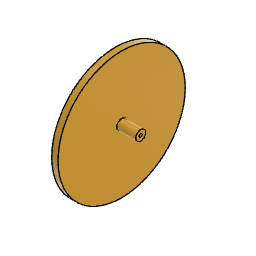
WaterMillWheelRimf3 (Autodesk Fusion 360 design; units mm, degrees)
Autodesk Fusion 360 part; units mm, degrees
sketch "Sketch1" plane through (0, 0, 0) normal (1, 0, 0) x (0, 1, 0)
  circle A0 centre (0, 0) radius 50
  dimension "d1" = 100
  constraint coincident A0.centre origin
  measures "d1" diameter of A0
extrude "Extrude1" add sketch "Sketch1" along normal blind 5
sketch "Sketch2" plane through (5, 0, 0) normal (1, 0, 0) x (0, 1, 0)
  circle A0 centre (0, 0) radius 50
  circle A1 centre (0, 0) radius 3.9375
  dimension "d4" = 7.875
  constraint concentric A0 A1
  measures "d4" diameter of A1
extrude "Extrude3" add sketch "Sketch2" along normal blind 15 contours A1
sketch "Sketch3" plane through (20, 0, 0) normal (1, 0, 0) x (0, 1, 0)
  circle A0 centre (0, 0) radius 3.9375
  circle A1 centre (0, 0) radius 1.2125
  dimension "d10" = 2.425
  constraint concentric A0 A1
  measures "d10" diameter of A1
extrude "Extrude4" cut sketch "Sketch3" against normal blind 12.125 contours A1
sketch "Sketch4" plane through (5, 0, 0) normal (1, 0, 0) x (0, 1, 0)
  circle A0 centre (0, 0) radius 50
  line L0 (-33.6779, 28.9291) -> (-27.8766, 32.541)
  line L1 (-27.8766, 32.541) -> (-24.8659, 32.541)
  spline S0 degree 3 poles (-24.8659, 32.541) (-24.773, 32.541) (-24.6881, 32.4676) (-24.6881, 32.363) knots 0 0 0 0 1 1 1 1
  spline S1 degree 3 poles (-24.6881, 32.363) (-24.6881, 32.2781) (-24.7268, 32.2432) (-24.773, 32.2162) knots 0 0 0 0 1 1 1 1
  line L2 (-24.773, 32.2162) -> (-27.6216, 30.5068)
  spline S2 degree 3 poles (-27.6216, 30.5068) (-27.8071, 30.3947) (-27.8728, 30.1742) (-27.8728, 30.008) knots 0 0 0 0 1 1 1 1
  line L3 (-27.8728, 30.008) -> (-27.8766, 28.9291)
  line L4 (-27.8766, 28.9291) -> (-24.2551, 28.9291)
  line L5 (-24.2551, 28.9291) -> (-24.2551, 35.1902)
  spline S3 degree 3 poles (-24.2551, 35.1902) (-24.2551, 35.31) (-24.348, 35.4144) (-24.4871, 35.4144) knots 0 0 0 0 1 1 1 1
  line L6 (-24.4871, 35.4144) -> (-27.9423, 35.4144)
  line L7 (-27.9423, 35.4144) -> (-33.7281, 31.8179)
  line L8 (-33.7281, 31.8179) -> (-33.7281, 28.9291)
  line L9 (-33.7281, 28.9291) -> (-33.6779, 28.9291)
  line L10 (13.8915, 28.9289) -> (19.1092, 28.9289)
  line L11 (19.1092, 28.9289) -> (19.1092, 30.3328)
  line L12 (19.1092, 30.3328) -> (15.5457, 30.3328)
  line L13 (15.5457, 30.3328) -> (15.5457, 31.5083)
  line L14 (15.5457, 31.5083) -> (18.4135, 31.5083)
  line L15 (18.4135, 31.5083) -> (18.4135, 32.9161)
  line L16 (18.4135, 32.9161) -> (15.5457, 32.9161)
  line L17 (15.5457, 32.9161) -> (15.5457, 34.0104)
  line L18 (15.5457, 34.0104) -> (19.1092, 34.0104)
  line L19 (19.1092, 34.0104) -> (19.1092, 35.4144)
  line L20 (19.1092, 35.4144) -> (13.8915, 35.4144)
  line L21 (13.8915, 35.4144) -> (13.8915, 28.9289)
  line L22 (-18.8945, 35.4144) -> (-21.3798, 28.9289)
  line L23 (-21.3798, 28.9289) -> (-19.6714, 28.9289)
  line L24 (-19.6714, 28.9289) -> (-19.2386, 30.1433)
  line L25 (-19.2386, 30.1433) -> (-16.4635, 30.1433)
  line L26 (-16.4635, 30.1433) -> (-16.0384, 28.9289)
  line L27 (-16.0384, 28.9289) -> (-14.2721, 28.9289)
  line L28 (-14.2721, 28.9289) -> (-16.7881, 35.4144)
  line L29 (-16.7881, 35.4144) -> (-18.8945, 35.4144)
  line L30 (-18.7477, 31.5238) -> (-17.8394, 34.0646)
  line L31 (-17.8394, 34.0646) -> (-16.9467, 31.5238)
  line L32 (-16.9467, 31.5238) -> (-18.7477, 31.5238)
  line L33 (-7.1839, 34.0104) -> (-5.093, 34.0104)
  line L34 (-5.093, 34.0104) -> (-5.093, 28.9289)
  line L35 (-5.093, 28.9289) -> (-3.4426, 28.9289)
  line L36 (-3.4426, 28.9289) -> (-3.4426, 34.0104)
  line L37 (-3.4426, 34.0104) -> (-1.3594, 34.0104)
  line L38 (-1.3594, 34.0104) -> (-1.3594, 35.4144)
  line L39 (-1.3594, 35.4144) -> (-7.1839, 35.4144)
  line L40 (-7.1839, 35.4144) -> (-7.1839, 34.0104)
  spline S4 degree 3 poles (-9.5878, 31.4272) (-9.5878, 30.584) (-10.1057, 30.2437) (-10.9908, 30.2437) knots 0 0 0 0 1 1 1 1
  spline S5 degree 3 poles (-10.9908, 30.2437) (-11.8488, 30.2437) (-12.4092, 30.5995) (-12.4092, 31.4272) knots 0 0 0 0 1 1 1 1
  line L41 (-12.4092, 31.4272) -> (-12.4092, 35.4376)
  line L42 (-12.4092, 35.4376) -> (-14.0634, 35.4376)
  line L43 (-14.0634, 35.4376) -> (-14.0634, 31.2377)
  spline S6 degree 3 poles (-14.0634, 31.2377) (-14.0634, 29.366) (-12.3937, 28.782) (-10.9947, 28.782) knots 0 0 0 0 1 1 1 1
  spline S7 degree 3 poles (-10.9947, 28.782) (-9.6033, 28.782) (-7.9414, 29.366) (-7.9414, 31.2377) knots 0 0 0 0 1 1 1 1
  line L44 (-7.9414, 31.2377) -> (-7.9414, 35.4376)
  line L45 (-7.9414, 35.4376) -> (-9.5955, 35.4376)
  line L46 (-9.5955, 35.4376) -> (-9.5955, 31.4272)
  line L47 (-9.5955, 31.4272) -> (-9.5878, 31.4272)
  line L48 (32.7484, 35.4144) -> (30.7811, 35.4144)
  line L49 (30.7811, 35.4144) -> (28.4237, 32.7807)
  line L50 (28.4237, 32.7807) -> (28.4237, 35.4144)
  line L51 (28.4237, 35.4144) -> (26.7693, 35.4144)
  line L52 (26.7693, 35.4144) -> (26.7771, 28.9289)
  line L53 (26.7771, 28.9289) -> (28.4237, 28.9289)
  line L54 (28.4237, 28.9289) -> (28.4237, 31.3923)
  line L55 (28.4237, 31.3923) -> (30.6575, 28.9289)
  line L56 (30.6575, 28.9289) -> (32.7484, 28.9289)
  line L57 (32.7484, 28.9289) -> (29.7338, 32.131)
  line L58 (29.7338, 32.131) -> (32.7484, 35.4144)
  line L59 (10.0033, 35.4144) -> (6.9732, 35.4144)
  line L60 (6.9732, 35.4144) -> (6.9732, 28.9289)
  line L61 (6.9732, 28.9289) -> (10.0033, 28.9289)
  spline S8 degree 3 poles (10.0033, 28.9289) (12.3262, 28.9289) (12.9678, 29.7952) (12.9678, 32.2199) knots 0 0 0 0 1 1 1 1
  spline S9 degree 3 poles (12.9678, 32.2199) (12.9678, 34.4978) (12.3532, 35.4144) (10.0033, 35.4144) knots 0 0 0 0 1 1 1 1
  line L62 (9.9377, 30.3328) -> (8.6236, 30.3328)
  line L63 (8.6236, 30.3328) -> (8.6236, 34.0104)
  line L64 (8.6236, 34.0104) -> (9.9377, 34.0104)
  spline S10 degree 3 poles (9.9377, 34.0104) (10.9735, 34.0104) (11.2827, 33.7283) (11.2827, 32.2199) knots 0 0 0 0 1 1 1 1
  spline S11 degree 3 poles (11.2827, 32.2199) (11.2827, 30.8432) (10.9348, 30.3328) (9.9377, 30.3328) knots 0 0 0 0 1 1 1 1
  line L65 (24.1065, 32.7458) -> (22.5992, 32.9161)
  spline S12 degree 3 poles (22.5992, 32.9161) (21.7179, 33.0127) (21.4976, 33.2332) (21.4976, 33.531) knots 0 0 0 0 1 1 1 1
  spline S13 degree 3 poles (21.4976, 33.531) (21.4976, 33.8636) (21.9499, 34.1613) (22.8349, 34.1613) knots 0 0 0 0 1 1 1 1
  spline S14 degree 3 poles (22.8349, 34.1613) (23.6852, 34.1613) (24.1297, 33.8442) (24.2109, 33.3685) knots 0 0 0 0 1 1 1 1
  line L66 (24.2109, 33.3685) -> (25.8303, 33.3685)
  spline S15 degree 3 poles (25.8303, 33.3685) (25.7489, 34.7415) (24.6012, 35.5922) (22.9238, 35.5922) knots 0 0 0 0 1 1 1 1
  spline S16 degree 3 poles (22.9238, 35.5922) (20.9295, 35.5922) (19.9286, 34.7994) (19.9286, 33.3955) knots 0 0 0 0 1 1 1 1
  spline S17 degree 3 poles (19.9286, 33.3955) (19.9286, 32.2547) (20.5933, 31.7171) (21.9691, 31.5703) knots 0 0 0 0 1 1 1 1
  line L67 (21.9691, 31.5703) -> (23.4997, 31.4077)
  spline S18 degree 3 poles (23.4997, 31.4077) (24.0833, 31.3421) (24.35, 31.1178) (24.35, 30.8239) knots 0 0 0 0 1 1 1 1
  spline S19 degree 3 poles (24.35, 30.8239) (24.35, 30.4914) (23.9596, 30.1935) (23.0204, 30.1935) knots 0 0 0 0 1 1 1 1
  spline S20 degree 3 poles (23.0204, 30.1935) (21.9344, 30.1935) (21.4976, 30.4681) (21.4242, 31.0212) knots 0 0 0 0 1 1 1 1
  line L68 (21.4242, 31.0212) -> (19.8357, 31.0212)
  spline S21 degree 3 poles (19.8357, 31.0212) (19.9091, 29.5283) (20.8793, 28.7665) (22.9625, 28.7665) knots 0 0 0 0 1 1 1 1
  spline S22 degree 3 poles (22.9625, 28.7665) (24.8639, 28.7665) (25.9267, 29.6018) (25.9267, 30.8587) knots 0 0 0 0 1 1 1 1
  spline S23 degree 3 poles (25.9267, 30.8587) (25.9267, 31.953) (25.2969, 32.6105) (24.1065, 32.7458) knots 0 0 0 0 1 1 1 1
  spline S24 degree 3 poles (2.4861, 35.5922) (0.1285, 35.5922) (-1.0927, 34.142) (-1.0927, 32.189) knots 0 0 0 0 1 1 1 1
  spline S25 degree 3 poles (-1.0927, 32.189) (-1.0927, 30.2282) (0.1285, 28.7703) (2.4861, 28.7703) knots 0 0 0 0 1 1 1 1
  spline S26 degree 3 poles (2.4861, 28.7703) (4.8515, 28.7703) (6.0729, 30.2282) (6.0729, 32.189) knots 0 0 0 0 1 1 1 1
  spline S27 degree 3 poles (6.0729, 32.189) (6.0767, 34.142) (4.8515, 35.5922) (2.4861, 35.5922) knots 0 0 0 0 1 1 1 1
  spline S28 degree 3 poles (2.4861, 30.2282) (1.2647, 30.2282) (0.5924, 30.9747) (0.5924, 32.189) knots 0 0 0 0 1 1 1 1
  spline S29 degree 3 poles (0.5924, 32.189) (0.5924, 33.3802) (1.2647, 34.1343) (2.4861, 34.1343) knots 0 0 0 0 1 1 1 1
  spline S30 degree 3 poles (2.4861, 34.1343) (3.719, 34.1343) (4.38, 33.3802) (4.38, 32.189) knots 0 0 0 0 1 1 1 1
  spline S31 degree 3 poles (4.38, 32.189) (4.3838, 30.9708) (3.719, 30.2282) (2.4861, 30.2282) knots 0 0 0 0 1 1 1 1
extrude "Extrude5" cut sketch "Sketch4" along normal blind 1 contours L0 L1 S0 S1 L2 S2 L3 L4 L5 S3 L6 L7 L8 L9 | L10 L11 L12 L13 L14 L15 L16 L17 L18 L19 L20 L21 | L22 L23 L24 L25 L26 L27 L28 L29 | L33 L34 L35 L36 L37 L38 L39 L40 | S4 S5 L41 L42 L43 S6 S7 L44 L45 L46 L47 | L48 L49 L50 L51 L52 L53 L54 L55 L56 L57 L58 | L59 L60 L61 S8 S9 | L65 S12 S13 S14 L66 S15 S16 S17 L67 S18 S19 S20 L68 S21 S22 S23 | S24 S25 S26 S27
sketch "Sketch5" plane through (5, 0, 0) normal (1, 0, 0) x (0, 1, 0)
  circle A0 centre (0, 0) radius 50
  circle A1 centre (0, 0) radius 3.9375
  spline S0 degree 3 poles (6.2324, -42.9698) (7.0803, -42.8865) (7.5571, -42.7606) (8.0991, -42.484) knots 0 0 0 0 1 1 1 1
  spline S1 degree 3 poles (8.0991, -42.484) (8.5579, -42.2478) (9.0099, -41.7778) (9.2573, -41.2785) knots 0 0 0 0 1 1 1 1
  spline S2 degree 3 poles (9.2573, -41.2785) (9.3293, -41.1301) (9.4327, -40.831) (9.4485, -40.723) knots 0 0 0 0 1 1 1 1
  spline S3 degree 3 poles (9.4485, -40.723) (9.453, -40.6871) (9.4574, -40.6556) (9.4597, -40.6556) knots 0 0 0 0 1 1 1 1
  spline S4 degree 3 poles (9.4597, -40.6556) (9.4619, -40.6556) (9.4664, -40.6263) (9.4709, -40.5881) knots 0 0 0 0 1 1 1 1
  spline S5 degree 3 poles (9.4709, -40.5881) (9.4732, -40.5521) (9.4889, -40.4352) (9.5047, -40.3295) knots 0 0 0 0 1 1 1 1
  spline S6 degree 3 poles (9.5047, -40.3295) (9.5429, -40.0619) (9.5384, -39.4276) (9.4934, -39.1038) knots 0 0 0 0 1 1 1 1
  spline S7 degree 3 poles (9.4934, -39.1038) (9.4732, -38.9554) (9.4552, -38.7957) (9.4574, -38.7507) knots 0 0 0 0 1 1 1 1
  spline S8 degree 3 poles (9.4574, -38.7507) (9.4574, -38.7035) (9.4462, -38.6608) (9.435, -38.654) knots 0 0 0 0 1 1 1 1
  spline S9 degree 3 poles (9.435, -38.654) (9.4237, -38.645) (9.4192, -38.6315) (9.426, -38.6203) knots 0 0 0 0 1 1 1 1
  spline S10 degree 3 poles (9.426, -38.6203) (9.4327, -38.609) (9.426, -38.5528) (9.4147, -38.4921) knots 0 0 0 0 1 1 1 1
  line L0 (9.4147, -38.4921) -> (9.39, -38.3796)
  line L1 (9.39, -38.3796) -> (9.1718, -38.3526)
  spline S11 degree 3 poles (9.1718, -38.3526) (8.4657, -38.2627) (7.5346, -38.076) (7.0443, -37.9298) knots 0 0 0 0 1 1 1 1
  spline S12 degree 3 poles (7.0443, -37.9298) (7.0196, -37.9231) (7.0601, -37.9658) (7.1343, -38.0243) knots 0 0 0 0 1 1 1 1
  spline S13 degree 3 poles (7.1343, -38.0243) (7.6313, -38.4246) (7.9956, -38.9351) (8.1688, -39.4861) knots 0 0 0 0 1 1 1 1
  spline S14 degree 3 poles (8.1688, -39.4861) (8.2295, -39.675) (8.234, -39.7133) (8.234, -40.0708) knots 0 0 0 0 1 1 1 1
  spline S15 degree 3 poles (8.234, -40.0708) (8.234, -40.4284) (8.2295, -40.4667) (8.1688, -40.6556) knots 0 0 0 0 1 1 1 1
  spline S16 degree 3 poles (8.1688, -40.6556) (8.0563, -41.0177) (7.8697, -41.373) (7.6943, -41.5642) knots 0 0 0 0 1 1 1 1
  spline S17 degree 3 poles (7.6943, -41.5642) (7.4469, -41.834) (7.0061, -42.0319) (6.4888, -42.1084) knots 0 0 0 0 1 1 1 1
  spline S18 degree 3 poles (6.4888, -42.1084) (6.1807, -42.1534) (5.6005, -42.1219) (5.2069, -42.0409) knots 0 0 0 0 1 1 1 1
  spline S19 degree 3 poles (5.2069, -42.0409) (4.6627, -41.9285) (3.97, -41.6946) (3.437, -41.4427) knots 0 0 0 0 1 1 1 1
  line L2 (3.437, -41.4427) -> (3.2301, -41.3438)
  line L3 (3.2301, -41.3438) -> (3.2301, -41.9937)
  line L4 (3.2301, -41.9937) -> (3.2301, -42.6437)
  line L5 (3.2301, -42.6437) -> (3.3245, -42.6706)
  spline S20 degree 3 poles (3.3245, -42.6706) (3.6484, -42.7584) (4.3028, -42.8731) (4.7819, -42.927) knots 0 0 0 0 1 1 1 1
  spline S21 degree 3 poles (4.7819, -42.927) (5.0697, -42.9608) (6.0413, -42.99) (6.2324, -42.9698) knots 0 0 0 0 1 1 1 1
  line L6 (19.3956, -42.8213) -> (19.3888, -42.7021)
  line L7 (19.3888, -42.7021) -> (19.164, -42.6751)
  spline S22 degree 3 poles (19.164, -42.6751) (19.0403, -42.6616) (18.8648, -42.6437) (18.7726, -42.6347) knots 0 0 0 0 1 1 1 1
  spline S23 degree 3 poles (18.7726, -42.6347) (18.4825, -42.6122) (17.909, -42.4975) (17.2298, -42.3288) knots 0 0 0 0 1 1 1 1
  spline S24 degree 3 poles (17.2298, -42.3288) (16.8948, -42.2456) (16.8475, -42.2276) (16.8025, -42.1601) knots 0 0 0 0 1 1 1 1
  spline S25 degree 3 poles (16.8025, -42.1601) (16.7373, -42.0612) (16.7598, -41.9442) (16.8948, -41.6609) knots 0 0 0 0 1 1 1 1
  spline S26 degree 3 poles (16.8948, -41.6609) (17.0792, -41.2808) (17.5357, -40.28) (17.5447, -40.2395) knots 0 0 0 0 1 1 1 1
  spline S27 degree 3 poles (17.5447, -40.2395) (17.5537, -40.2035) (17.6594, -39.9674) (17.8686, -39.5311) knots 0 0 0 0 1 1 1 1
  spline S28 degree 3 poles (17.8686, -39.5311) (17.963, -39.3332) (18.5702, -38.0018) (18.5792, -37.9771) knots 0 0 0 0 1 1 1 1
  spline S29 degree 3 poles (18.5792, -37.9771) (18.5792, -37.9748) (18.7569, -37.9456) (18.9728, -37.9141) knots 0 0 0 0 1 1 1 1
  spline S30 degree 3 poles (18.9728, -37.9141) (19.5305, -37.8286) (20.4504, -37.6667) (21.0418, -37.552) knots 0 0 0 0 1 1 1 1
  spline S31 degree 3 poles (21.0418, -37.552) (21.5456, -37.4508) (21.6738, -37.4283) (21.739, -37.4261) knots 0 0 0 0 1 1 1 1
  spline S32 degree 3 poles (21.739, -37.4261) (21.9414, -37.4148) (23.8418, -36.9448) (24.359, -36.7784) knots 0 0 0 0 1 1 1 1
  spline S33 degree 3 poles (24.359, -36.7784) (24.5322, -36.7221) (24.4445, -36.7177) (24.1994, -36.7671) knots 0 0 0 0 1 1 1 1
  spline S34 degree 3 poles (24.1994, -36.7671) (24.0779, -36.7919) (23.97, -36.8009) (23.8598, -36.7896) knots 0 0 0 0 1 1 1 1
  spline S35 degree 3 poles (23.8598, -36.7896) (23.7248, -36.7784) (23.6079, -36.7941) (23.1626, -36.8773) knots 0 0 0 0 1 1 1 1
  spline S36 degree 3 poles (23.1626, -36.8773) (21.6558, -37.1562) (20.1063, -37.3384) (19.2292, -37.3384) knots 0 0 0 0 1 1 1 1
  spline S37 degree 3 poles (19.2292, -37.3384) (18.9458, -37.3384) (18.9053, -37.3339) (18.9053, -37.3024) knots 0 0 0 0 1 1 1 1
  spline S38 degree 3 poles (18.9053, -37.3024) (18.9053, -37.2664) (19.3079, -36.3601) (19.3641, -36.2701) knots 0 0 0 0 1 1 1 1
  spline S39 degree 3 poles (19.3641, -36.2701) (19.4023, -36.2094) (19.6272, -35.7169) (19.6362, -35.6741) knots 0 0 0 0 1 1 1 1
  spline S40 degree 3 poles (19.6362, -35.6741) (19.6452, -35.6337) (20.1647, -34.4957) (20.2412, -34.3472) knots 0 0 0 0 1 1 1 1
  spline S41 degree 3 poles (20.2412, -34.3472) (20.3042, -34.2258) (20.6145, -33.5444) (20.6145, -33.5264) knots 0 0 0 0 1 1 1 1
  spline S42 degree 3 poles (20.6145, -33.5264) (20.6145, -33.5084) (21.0598, -32.5346) (21.1565, -32.3412) knots 0 0 0 0 1 1 1 1
  line L8 (21.1565, -32.3412) -> (21.2442, -32.1658)
  line L9 (21.2442, -32.1658) -> (20.7427, -32.1658)
  line L10 (20.7427, -32.1658) -> (20.2412, -32.1658)
  line L11 (20.2412, -32.1658) -> (20.0883, -32.4874)
  spline S43 degree 3 poles (20.0883, -32.4874) (20.0028, -32.6628) (19.8634, -32.9641) (19.7779, -33.1553) knots 0 0 0 0 1 1 1 1
  spline S44 degree 3 poles (19.7779, -33.1553) (19.4023, -33.9874) (19.3191, -34.1718) (19.1977, -34.426) knots 0 0 0 0 1 1 1 1
  spline S45 degree 3 poles (19.1977, -34.426) (19.0403, -34.7543) (18.6782, -35.5414) (18.6354, -35.6516) knots 0 0 0 0 1 1 1 1
  spline S46 degree 3 poles (18.6354, -35.6516) (18.6175, -35.6944) (18.5095, -35.9328) (18.3926, -36.1802) knots 0 0 0 0 1 1 1 1
  spline S47 degree 3 poles (18.3926, -36.1802) (18.2779, -36.4275) (18.1047, -36.7986) (18.0102, -37.0055) knots 0 0 0 0 1 1 1 1
  spline S48 degree 3 poles (18.0102, -37.0055) (17.8416, -37.3698) (17.8348, -37.3833) (17.7584, -37.3991) knots 0 0 0 0 1 1 1 1
  spline S49 degree 3 poles (17.7584, -37.3991) (17.6302, -37.4283) (15.5206, -37.4193) (14.9696, -37.3878) knots 0 0 0 0 1 1 1 1
  spline S50 degree 3 poles (14.9696, -37.3878) (14.5693, -37.3631) (14.4501, -37.3496) (14.3962, -37.3181) knots 0 0 0 0 1 1 1 1
  spline S51 degree 3 poles (14.3962, -37.3181) (14.3399, -37.2866) (14.2995, -37.2124) (14.1533, -36.8773) knots 0 0 0 0 1 1 1 1
  spline S52 degree 3 poles (14.1533, -36.8773) (13.8991, -36.2903) (13.5056, -35.3503) (13.4966, -35.3031) knots 0 0 0 0 1 1 1 1
  spline S53 degree 3 poles (13.4966, -35.3031) (13.4921, -35.2896) (13.4269, -35.1321) (13.3504, -34.9545) knots 0 0 0 0 1 1 1 1
  spline S54 degree 3 poles (13.3504, -34.9545) (13.2739, -34.7746) (13.0918, -34.345) (12.9478, -33.9987) knots 0 0 0 0 1 1 1 1
  spline S55 degree 3 poles (12.9478, -33.9987) (12.8017, -33.6523) (12.651, -33.3037) (12.615, -33.2228) knots 0 0 0 0 1 1 1 1
  spline S56 degree 3 poles (12.615, -33.2228) (12.5408, -33.0586) (12.4845, -32.9259) (12.4845, -32.9057) knots 0 0 0 0 1 1 1 1
  spline S57 degree 3 poles (12.4845, -32.9057) (12.4845, -32.8989) (12.4238, -32.746) (12.3496, -32.5661) knots 0 0 0 0 1 1 1 1
  line L12 (12.3496, -32.5661) -> (12.2147, -32.24)
  line L13 (12.2147, -32.24) -> (11.965, -32.2265)
  spline S58 degree 3 poles (11.965, -32.2265) (11.5962, -32.2085) (11.3353, -32.123) (11.034, -31.9184) knots 0 0 0 0 1 1 1 1
  spline S59 degree 3 poles (11.034, -31.9184) (10.8293, -31.7767) (10.5167, -31.617) (10.5167, -31.653) knots 0 0 0 0 1 1 1 1
  spline S60 degree 3 poles (10.5167, -31.653) (10.5167, -31.671) (10.528, -31.6957) (10.5437, -31.7115) knots 0 0 0 0 1 1 1 1
  spline S61 degree 3 poles (10.5437, -31.7115) (10.5594, -31.7272) (10.5639, -31.7385) (10.5549, -31.7385) knots 0 0 0 0 1 1 1 1
  spline S62 degree 3 poles (10.5549, -31.7385) (10.5414, -31.7385) (10.6449, -31.9948) (10.7416, -32.1995) knots 0 0 0 0 1 1 1 1
  spline S63 degree 3 poles (10.7416, -32.1995) (10.7641, -32.249) (10.899, -32.5683) (11.043, -32.9079) knots 0 0 0 0 1 1 1 1
  spline S64 degree 3 poles (11.043, -32.9079) (11.1846, -33.2475) (11.3623, -33.6726) (11.4388, -33.8525) knots 0 0 0 0 1 1 1 1
  spline S65 degree 3 poles (11.4388, -33.8525) (11.5152, -34.0324) (11.5805, -34.1943) (11.585, -34.2123) knots 0 0 0 0 1 1 1 1
  spline S66 degree 3 poles (11.585, -34.2123) (11.5917, -34.2528) (12.0258, -35.2963) (12.1022, -35.4605) knots 0 0 0 0 1 1 1 1
  spline S67 degree 3 poles (12.1022, -35.4605) (12.1809, -35.6314) (12.5655, -36.558) (12.5745, -36.5985) knots 0 0 0 0 1 1 1 1
  spline S68 degree 3 poles (12.5745, -36.5985) (12.579, -36.6187) (12.6285, -36.7446) (12.6847, -36.8796) knots 0 0 0 0 1 1 1 1
  spline S69 degree 3 poles (12.6847, -36.8796) (12.7927, -37.1337) (12.8039, -37.1809) (12.7634, -37.1809) knots 0 0 0 0 1 1 1 1
  spline S70 degree 3 poles (12.7634, -37.1809) (12.7499, -37.1809) (12.489, -37.1495) (12.1832, -37.1112) knots 0 0 0 0 1 1 1 1
  spline S71 degree 3 poles (12.1832, -37.1112) (11.3758, -37.0123) (10.5729, -36.8818) (9.8195, -36.7289) knots 0 0 0 0 1 1 1 1
  spline S72 degree 3 poles (9.8195, -36.7289) (9.4552, -36.6547) (9.0999, -36.5827) (9.0324, -36.5692) knots 0 0 0 0 1 1 1 1
  spline S73 degree 3 poles (9.0324, -36.5692) (8.83, -36.531) (8.0968, -36.3331) (7.7955, -36.2386) knots 0 0 0 0 1 1 1 1
  spline S74 degree 3 poles (7.7955, -36.2386) (7.1455, -36.034) (6.174, -35.6404) (5.8051, -35.4357) knots 0 0 0 0 1 1 1 1
  spline S75 degree 3 poles (5.8051, -35.4357) (4.9258, -34.9455) (4.3186, -34.4102) (4.042, -33.875) knots 0 0 0 0 1 1 1 1
  spline S76 degree 3 poles (4.042, -33.875) (3.9003, -33.6006) (3.8733, -33.4949) (3.8913, -33.2745) knots 0 0 0 0 1 1 1 1
  spline S77 degree 3 poles (3.8913, -33.2745) (3.9318, -32.782) (4.1432, -32.3254) (4.5435, -31.8666) knots 0 0 0 0 1 1 1 1
  spline S78 degree 3 poles (4.5435, -31.8666) (5.0135, -31.3291) (6.012, -30.6814) (7.0128, -30.2631) knots 0 0 0 0 1 1 1 1
  spline S79 degree 3 poles (7.0128, -30.2631) (7.1568, -30.2047) (7.2737, -30.1529) (7.2715, -30.1484) knots 0 0 0 0 1 1 1 1
  spline S80 degree 3 poles (7.2715, -30.1484) (7.2647, -30.1417) (7.1568, -30.1709) (6.5473, -30.3464) knots 0 0 0 0 1 1 1 1
  spline S81 degree 3 poles (6.5473, -30.3464) (5.6207, -30.614) (4.6694, -31.0143) (4.1297, -31.3674) knots 0 0 0 0 1 1 1 1
  spline S82 degree 3 poles (4.1297, -31.3674) (4.0262, -31.4348) (3.9273, -31.4911) (3.9115, -31.4911) knots 0 0 0 0 1 1 1 1
  spline S83 degree 3 poles (3.9115, -31.4911) (3.8958, -31.4911) (3.8823, -31.5023) (3.8823, -31.5136) knots 0 0 0 0 1 1 1 1
  spline S84 degree 3 poles (3.8823, -31.5136) (3.8823, -31.5271) (3.8733, -31.5361) (3.8598, -31.5361) knots 0 0 0 0 1 1 1 1
  spline S85 degree 3 poles (3.8598, -31.5361) (3.8485, -31.5361) (3.8193, -31.5495) (3.7991, -31.5675) knots 0 0 0 0 1 1 1 1
  spline S86 degree 3 poles (3.7991, -31.5675) (3.7766, -31.5855) (3.6574, -31.68) (3.5314, -31.7789) knots 0 0 0 0 1 1 1 1
  spline S87 degree 3 poles (3.5314, -31.7789) (3.2728, -31.9858) (2.9872, -32.2805) (2.832, -32.4986) knots 0 0 0 0 1 1 1 1
  spline S88 degree 3 poles (2.832, -32.4986) (2.7735, -32.5818) (2.7196, -32.6538) (2.7106, -32.6605) knots 0 0 0 0 1 1 1 1
  spline S89 degree 3 poles (2.7106, -32.6605) (2.6521, -32.7055) (2.4317, -33.2565) (2.4452, -33.3262) knots 0 0 0 0 1 1 1 1
  spline S90 degree 3 poles (2.4452, -33.3262) (2.4474, -33.3375) (2.4474, -33.351) (2.4429, -33.3577) knots 0 0 0 0 1 1 1 1
  spline S91 degree 3 poles (2.4429, -33.3577) (2.4384, -33.3712) (2.4384, -33.7468) (2.4429, -33.7625) knots 0 0 0 0 1 1 1 1
  spline S92 degree 3 poles (2.4429, -33.7625) (2.4452, -33.7693) (2.4497, -33.7985) (2.4564, -33.83) knots 0 0 0 0 1 1 1 1
  spline S93 degree 3 poles (2.4564, -33.83) (2.4699, -33.9154) (2.6296, -34.2258) (2.7623, -34.426) knots 0 0 0 0 1 1 1 1
  spline S94 degree 3 poles (2.7623, -34.426) (2.895, -34.6239) (3.2886, -35.0444) (3.5202, -35.2333) knots 0 0 0 0 1 1 1 1
  spline S95 degree 3 poles (3.5202, -35.2333) (3.6551, -35.3435) (3.952, -35.5459) (4.3141, -35.7753) knots 0 0 0 0 1 1 1 1
  spline S96 degree 3 poles (4.3141, -35.7753) (4.584, -35.9463) (5.5285, -36.3916) (5.6927, -36.4253) knots 0 0 0 0 1 1 1 1
  spline S97 degree 3 poles (5.6927, -36.4253) (5.7174, -36.432) (5.9041, -36.4973) (6.1065, -36.5737) knots 0 0 0 0 1 1 1 1
  spline S98 degree 3 poles (6.1065, -36.5737) (6.3089, -36.6502) (6.6935, -36.7761) (6.9611, -36.8548) knots 0 0 0 0 1 1 1 1
  spline S99 degree 3 poles (6.9611, -36.8548) (7.2287, -36.9358) (7.4761, -37.01) (7.5143, -37.0213) knots 0 0 0 0 1 1 1 1
  spline S100 degree 3 poles (7.5143, -37.0213) (7.719, -37.0887) (9.1426, -37.4171) (9.3203, -37.4396) knots 0 0 0 0 1 1 1 1
  spline S101 degree 3 poles (9.3203, -37.4396) (9.3652, -37.4463) (9.444, -37.4576) (9.4934, -37.4621) knots 0 0 0 0 1 1 1 1
  spline S102 degree 3 poles (9.4934, -37.4621) (9.5429, -37.4688) (9.7453, -37.5048) (9.9432, -37.5408) knots 0 0 0 0 1 1 1 1
  spline S103 degree 3 poles (9.9432, -37.5408) (10.8158, -37.6982) (12.3564, -37.9029) (13.0468, -37.9501) knots 0 0 0 0 1 1 1 1
  line L14 (13.0468, -37.9501) -> (13.1367, -37.9568)
  line L15 (13.1367, -37.9568) -> (13.2829, -38.3077)
  spline S104 degree 3 poles (13.2829, -38.3077) (13.3639, -38.5011) (13.4493, -38.7035) (13.4718, -38.7575) knots 0 0 0 0 1 1 1 1
  spline S105 degree 3 poles (13.4718, -38.7575) (13.4966, -38.8114) (13.5348, -38.8991) (13.5573, -38.9531) knots 0 0 0 0 1 1 1 1
  spline S106 degree 3 poles (13.5573, -38.9531) (13.582, -39.0071) (13.6045, -39.0678) (13.609, -39.0881) knots 0 0 0 0 1 1 1 1
  spline S107 degree 3 poles (13.609, -39.0881) (13.6158, -39.1263) (14.1263, -40.37) (14.2095, -40.5544) knots 0 0 0 0 1 1 1 1
  spline S108 degree 3 poles (14.2095, -40.5544) (14.2905, -40.7275) (14.5896, -41.463) (14.5986, -41.5057) knots 0 0 0 0 1 1 1 1
  spline S109 degree 3 poles (14.5986, -41.5057) (14.6031, -41.5259) (14.6143, -41.5574) (14.6256, -41.5732) knots 0 0 0 0 1 1 1 1
  spline S110 degree 3 poles (14.6256, -41.5732) (14.6346, -41.5866) (14.6435, -41.6114) (14.6458, -41.6226) knots 0 0 0 0 1 1 1 1
  spline S111 degree 3 poles (14.6458, -41.6226) (14.6503, -41.6429) (14.8055, -42.0229) (15.0933, -42.7021) knots 0 0 0 0 1 1 1 1
  line L16 (15.0933, -42.7021) -> (15.1878, -42.927)
  line L17 (15.1878, -42.927) -> (17.2951, -42.9338)
  line L18 (17.2951, -42.9338) -> (19.4023, -42.9383)
  line L19 (19.4023, -42.9383) -> (19.3956, -42.8213)
  spline S112 degree 3 poles (15.9682, -41.301) (15.9457, -41.2853) (15.8085, -40.9682) (15.3295, -39.8235) knots 0 0 0 0 1 1 1 1
  spline S113 degree 3 poles (15.3295, -39.8235) (15.1855, -39.4771) (15.0439, -39.1443) (15.0146, -39.0813) knots 0 0 0 0 1 1 1 1
  spline S114 degree 3 poles (15.0146, -39.0813) (14.9854, -39.0206) (14.9629, -38.9554) (14.9629, -38.9419) knots 0 0 0 0 1 1 1 1
  spline S115 degree 3 poles (14.9629, -38.9419) (14.9629, -38.9261) (14.9562, -38.9126) (14.9472, -38.9126) knots 0 0 0 0 1 1 1 1
  spline S116 degree 3 poles (14.9472, -38.9126) (14.9382, -38.9126) (14.9314, -38.8991) (14.9314, -38.8856) knots 0 0 0 0 1 1 1 1
  spline S117 degree 3 poles (14.9314, -38.8856) (14.9314, -38.8699) (14.8639, -38.6922) (14.7785, -38.4921) knots 0 0 0 0 1 1 1 1
  spline S118 degree 3 poles (14.7785, -38.4921) (14.6863, -38.2694) (14.6323, -38.1143) (14.6413, -38.0895) knots 0 0 0 0 1 1 1 1
  spline S119 degree 3 poles (14.6413, -38.0895) (14.6548, -38.0558) (14.6818, -38.0535) (14.8977, -38.0693) knots 0 0 0 0 1 1 1 1
  spline S120 degree 3 poles (14.8977, -38.0693) (15.0304, -38.0783) (15.6601, -38.0895) (16.2965, -38.0918) knots 0 0 0 0 1 1 1 1
  spline S121 degree 3 poles (16.2965, -38.0918) (17.1039, -38.0963) (17.4547, -38.1053) (17.4615, -38.1233) knots 0 0 0 0 1 1 1 1
  spline S122 degree 3 poles (17.4615, -38.1233) (17.466, -38.1367) (17.4165, -38.2604) (17.3535, -38.3999) knots 0 0 0 0 1 1 1 1
  spline S123 degree 3 poles (17.3535, -38.3999) (17.2883, -38.5393) (17.2343, -38.6697) (17.2298, -38.6877) knots 0 0 0 0 1 1 1 1
  spline S124 degree 3 poles (17.2298, -38.6877) (17.2254, -38.708) (17.1511, -38.8789) (17.0612, -39.0701) knots 0 0 0 0 1 1 1 1
  spline S125 degree 3 poles (17.0612, -39.0701) (16.6474, -39.9651) (16.2223, -40.9052) (16.2223, -40.9322) knots 0 0 0 0 1 1 1 1
  spline S126 degree 3 poles (16.2223, -40.9322) (16.2223, -40.9457) (16.2111, -40.9592) (16.1998, -40.9592) knots 0 0 0 0 1 1 1 1
  spline S127 degree 3 poles (16.1998, -40.9592) (16.1863, -40.9592) (16.1818, -40.9659) (16.1908, -40.9727) knots 0 0 0 0 1 1 1 1
  spline S128 degree 3 poles (16.1908, -40.9727) (16.2021, -40.9862) (16.0896, -41.2313) (16.0424, -41.292) knots 0 0 0 0 1 1 1 1
  spline S129 degree 3 poles (16.0424, -41.292) (16.0177, -41.3235) (16.0019, -41.3258) (15.9682, -41.301) knots 0 0 0 0 1 1 1 1
  spline S130 degree 3 poles (2.1506, -42.5582) (2.1506, -42.5222) (2.1258, -42.5155) (1.9527, -42.502) knots 0 0 0 0 1 1 1 1
  spline S131 degree 3 poles (1.9527, -42.502) (0.682, -42.4008) (-0.2311, -41.9892) (-0.5549, -41.3685) knots 0 0 0 0 1 1 1 1
  spline S132 degree 3 poles (-0.5549, -41.3685) (-0.5976, -41.2853) (-0.6449, -41.1773) (-0.6584, -41.1279) knots 0 0 0 0 1 1 1 1
  spline S133 degree 3 poles (-0.6584, -41.1279) (-0.6764, -41.0649) (-0.6831, -39.756) (-0.6831, -36.612) knots 0 0 0 0 1 1 1 1
  line L20 (-0.6831, -36.612) -> (-0.6831, -32.1882)
  line L21 (-0.6831, -32.1882) -> (-1.1149, -32.1927)
  line L22 (-1.1149, -32.1927) -> (-1.549, -32.1995)
  line L23 (-1.549, -32.1995) -> (-1.549, -37.064)
  spline S134 degree 3 poles (-1.549, -37.064) (-1.549, -41.4202) (-1.5535, -41.9262) (-1.5827, -41.9262) knots 0 0 0 0 1 1 1 1
  spline S135 degree 3 poles (-1.5827, -41.9262) (-1.6029, -41.9262) (-1.6344, -41.897) (-1.6547, -41.8633) knots 0 0 0 0 1 1 1 1
  spline S136 degree 3 poles (-1.6547, -41.8633) (-1.6771, -41.8273) (-1.9088, -41.4944) (-2.1719, -41.1211) knots 0 0 0 0 1 1 1 1
  spline S137 degree 3 poles (-2.1719, -41.1211) (-2.435, -40.7478) (-2.7881, -40.2485) (-2.9546, -40.0101) knots 0 0 0 0 1 1 1 1
  spline S138 degree 3 poles (-2.9546, -40.0101) (-3.121, -39.774) (-3.2739, -39.5626) (-3.2941, -39.5446) knots 0 0 0 0 1 1 1 1
  spline S139 degree 3 poles (-3.2941, -39.5446) (-3.3121, -39.5244) (-3.4178, -39.3827) (-3.5258, -39.2275) knots 0 0 0 0 1 1 1 1
  spline S140 degree 3 poles (-3.5258, -39.2275) (-3.6337, -39.0723) (-3.9508, -38.6203) (-4.232, -38.2222) knots 0 0 0 0 1 1 1 1
  spline S141 degree 3 poles (-4.232, -38.2222) (-4.5131, -37.8241) (-4.9246, -37.2394) (-5.1473, -36.9223) knots 0 0 0 0 1 1 1 1
  spline S142 degree 3 poles (-5.1473, -36.9223) (-5.3699, -36.6075) (-5.5588, -36.3488) (-5.5701, -36.3488) knots 0 0 0 0 1 1 1 1
  spline S143 degree 3 poles (-5.5701, -36.3488) (-5.5791, -36.3488) (-5.5858, -36.3331) (-5.5858, -36.3151) knots 0 0 0 0 1 1 1 1
  spline S144 degree 3 poles (-5.5858, -36.3151) (-5.5858, -36.2971) (-5.5971, -36.2814) (-5.6083, -36.2814) knots 0 0 0 0 1 1 1 1
  spline S145 degree 3 poles (-5.6083, -36.2814) (-5.6218, -36.2814) (-5.6308, -36.2656) (-5.6308, -36.2476) knots 0 0 0 0 1 1 1 1
  spline S146 degree 3 poles (-5.6308, -36.2476) (-5.6308, -36.2274) (-5.6466, -36.2071) (-5.6645, -36.2004) knots 0 0 0 0 1 1 1 1
  spline S147 degree 3 poles (-5.6645, -36.2004) (-5.6825, -36.1914) (-5.6983, -36.1757) (-5.6983, -36.1599) knots 0 0 0 0 1 1 1 1
  spline S148 degree 3 poles (-5.6983, -36.1599) (-5.6983, -36.1464) (-5.759, -36.052) (-5.831, -35.9485) knots 0 0 0 0 1 1 1 1
  line L24 (-5.831, -35.9485) -> (-5.9637, -35.7641)
  line L25 (-5.9637, -35.7641) -> (-6.0626, -35.9035)
  spline S149 degree 3 poles (-6.0626, -35.9035) (-6.1188, -35.9822) (-6.355, -36.3286) (-6.5866, -36.6749) knots 0 0 0 0 1 1 1 1
  spline S150 degree 3 poles (-6.5866, -36.6749) (-6.8205, -37.0213) (-7.0589, -37.3698) (-7.1174, -37.4508) knots 0 0 0 0 1 1 1 1
  spline S151 degree 3 poles (-7.1174, -37.4508) (-7.2321, -37.6082) (-7.9068, -38.5978) (-8.7569, -39.8572) knots 0 0 0 0 1 1 1 1
  spline S152 degree 3 poles (-8.7569, -39.8572) (-9.0447, -40.2845) (-9.2989, -40.6556) (-9.3236, -40.6826) knots 0 0 0 0 1 1 1 1
  spline S153 degree 3 poles (-9.3236, -40.6826) (-9.3483, -40.7096) (-9.5485, -40.9974) (-9.7666, -41.3235) knots 0 0 0 0 1 1 1 1
  spline S154 degree 3 poles (-9.7666, -41.3235) (-9.987, -41.6496) (-10.1827, -41.9172) (-10.2029, -41.9217) knots 0 0 0 0 1 1 1 1
  spline S155 degree 3 poles (-10.2029, -41.9217) (-10.2389, -41.9285) (-10.2412, -41.6001) (-10.2412, -37.0595) knots 0 0 0 0 1 1 1 1
  line L26 (-10.2412, -37.0595) -> (-10.2412, -32.1882)
  line L27 (-10.2412, -32.1882) -> (-10.9721, -32.1927)
  line L28 (-10.9721, -32.1927) -> (-11.703, -32.1995)
  line L29 (-11.703, -32.1995) -> (-11.703, -37.3946)
  line L30 (-11.703, -37.3946) -> (-11.703, -42.5897)
  line L31 (-11.703, -42.5897) -> (-10.6752, -42.5942)
  line L32 (-10.6752, -42.5942) -> (-9.6452, -42.5987)
  line L33 (-9.6452, -42.5987) -> (-9.2516, -42.0432)
  spline S156 degree 3 poles (-9.2516, -42.0432) (-8.4195, -40.8737) (-8.0529, -40.3632) (-8.0349, -40.3565) knots 0 0 0 0 1 1 1 1
  spline S157 degree 3 poles (-8.0349, -40.3565) (-8.0237, -40.352) (-8.0147, -40.334) (-8.0147, -40.3182) knots 0 0 0 0 1 1 1 1
  spline S158 degree 3 poles (-8.0147, -40.3182) (-8.0147, -40.3002) (-8.0012, -40.2778) (-7.9855, -40.2688) knots 0 0 0 0 1 1 1 1
  spline S159 degree 3 poles (-7.9855, -40.2688) (-7.945, -40.2418) (-7.7448, -39.9651) (-7.7448, -39.9337) knots 0 0 0 0 1 1 1 1
  spline S160 degree 3 poles (-7.7448, -39.9337) (-7.7448, -39.9202) (-7.7291, -39.9022) (-7.7111, -39.8932) knots 0 0 0 0 1 1 1 1
  spline S161 degree 3 poles (-7.7111, -39.8932) (-7.6931, -39.8864) (-7.6774, -39.8662) (-7.6774, -39.846) knots 0 0 0 0 1 1 1 1
  spline S162 degree 3 poles (-7.6774, -39.846) (-7.6774, -39.828) (-7.6684, -39.8122) (-7.6549, -39.8122) knots 0 0 0 0 1 1 1 1
  spline S163 degree 3 poles (-7.6549, -39.8122) (-7.6436, -39.8122) (-7.6324, -39.7987) (-7.6324, -39.7807) knots 0 0 0 0 1 1 1 1
  spline S164 degree 3 poles (-7.6324, -39.7807) (-7.6324, -39.7627) (-7.6166, -39.7447) (-7.5987, -39.7358) knots 0 0 0 0 1 1 1 1
  spline S165 degree 3 poles (-7.5987, -39.7358) (-7.5807, -39.729) (-7.5649, -39.7088) (-7.5649, -39.6908) knots 0 0 0 0 1 1 1 1
  spline S166 degree 3 poles (-7.5649, -39.6908) (-7.5649, -39.6728) (-7.5559, -39.6548) (-7.5447, -39.6503) knots 0 0 0 0 1 1 1 1
  spline S167 degree 3 poles (-7.5447, -39.6503) (-7.5289, -39.6435) (-7.1331, -39.097) (-6.5124, -38.2222) knots 0 0 0 0 1 1 1 1
  spline S168 degree 3 poles (-6.5124, -38.2222) (-6.4045, -38.0715) (-6.301, -37.9478) (-6.283, -37.9478) knots 0 0 0 0 1 1 1 1
  spline S169 degree 3 poles (-6.283, -37.9478) (-6.2493, -37.9478) (-6.1886, -38.0243) (-5.4059, -39.0476) knots 0 0 0 0 1 1 1 1
  spline S170 degree 3 poles (-5.4059, -39.0476) (-5.1923, -39.3264) (-5.0011, -39.5693) (-4.9809, -39.5873) knots 0 0 0 0 1 1 1 1
  spline S171 degree 3 poles (-4.9809, -39.5873) (-4.9606, -39.6053) (-4.9359, -39.639) (-4.9269, -39.6615) knots 0 0 0 0 1 1 1 1
  spline S172 degree 3 poles (-4.9269, -39.6615) (-4.9201, -39.6818) (-4.9022, -39.6998) (-4.8887, -39.6998) knots 0 0 0 0 1 1 1 1
  spline S173 degree 3 poles (-4.8887, -39.6998) (-4.8774, -39.6998) (-4.8662, -39.7155) (-4.8662, -39.7335) knots 0 0 0 0 1 1 1 1
  spline S174 degree 3 poles (-4.8662, -39.7335) (-4.8662, -39.7515) (-4.8459, -39.7785) (-4.8212, -39.7942) knots 0 0 0 0 1 1 1 1
  spline S175 degree 3 poles (-4.8212, -39.7942) (-4.7964, -39.81) (-4.7762, -39.837) (-4.7762, -39.8527) knots 0 0 0 0 1 1 1 1
  spline S176 degree 3 poles (-4.7762, -39.8527) (-4.7762, -39.8684) (-4.7605, -39.8864) (-4.7425, -39.8932) knots 0 0 0 0 1 1 1 1
  spline S177 degree 3 poles (-4.7425, -39.8932) (-4.7245, -39.9022) (-4.7087, -39.9202) (-4.7087, -39.9382) knots 0 0 0 0 1 1 1 1
  spline S178 degree 3 poles (-4.7087, -39.9382) (-4.7087, -39.9539) (-4.6907, -39.9786) (-4.6705, -39.9899) knots 0 0 0 0 1 1 1 1
  spline S179 degree 3 poles (-4.6705, -39.9899) (-4.648, -40.0034) (-4.639, -40.0146) (-4.648, -40.0146) knots 0 0 0 0 1 1 1 1
  spline S180 degree 3 poles (-4.648, -40.0146) (-4.6638, -40.0146) (-4.5671, -40.1428) (-4.4546, -40.2733) knots 0 0 0 0 1 1 1 1
  spline S181 degree 3 poles (-4.4546, -40.2733) (-4.4321, -40.298) (-4.4006, -40.334) (-4.3849, -40.352) knots 0 0 0 0 1 1 1 1
  spline S182 degree 3 poles (-4.3849, -40.352) (-4.3557, -40.3857) (-4.1308, -40.6758) (-3.1457, -41.9577) knots 0 0 0 0 1 1 1 1
  line L34 (-3.1457, -41.9577) -> (-2.6509, -42.5987)
  line L35 (-2.6509, -42.5987) -> (-0.2513, -42.6009)
  spline S183 degree 3 poles (-0.2513, -42.6009) (2.0854, -42.6009) (2.1506, -42.5987) (2.1506, -42.5582) knots 0 0 0 0 1 1 1 1
  line L36 (-12.5126, -42.511) -> (-12.5126, -42.421)
  line L37 (-12.5126, -42.421) -> (-12.6251, -42.421)
  spline S184 degree 3 poles (-12.6251, -42.421) (-12.9714, -42.421) (-13.6034, -42.3063) (-13.9272, -42.1849) knots 0 0 0 0 1 1 1 1
  spline S185 degree 3 poles (-13.9272, -42.1849) (-14.5479, -41.9532) (-14.8853, -41.6541) (-15.0472, -41.1953) knots 0 0 0 0 1 1 1 1
  line L38 (-15.0472, -41.1953) -> (-15.1102, -41.0154)
  line L39 (-15.1102, -41.0154) -> (-15.1169, -36.603)
  line L40 (-15.1169, -36.603) -> (-15.1214, -32.1882)
  line L41 (-15.1214, -32.1882) -> (-18.4026, -32.1882)
  line L42 (-18.4026, -32.1882) -> (-21.6839, -32.1882)
  line L43 (-21.6839, -32.1882) -> (-21.6974, -32.3749)
  spline S186 degree 3 poles (-21.6974, -32.3749) (-21.7131, -32.5683) (-21.7783, -33.9964) (-21.7783, -34.1066) knots 0 0 0 0 1 1 1 1
  spline S187 degree 3 poles (-21.7783, -34.1066) (-21.7783, -34.1628) (-21.7626, -34.1493) (-21.6389, -33.9852) knots 0 0 0 0 1 1 1 1
  spline S188 degree 3 poles (-21.6389, -33.9852) (-21.2678, -33.4926) (-20.7303, -33.0811) (-20.2378, -32.9124) knots 0 0 0 0 1 1 1 1
  spline S189 degree 3 poles (-20.2378, -32.9124) (-19.9117, -32.8022) (-19.8195, -32.7955) (-18.3712, -32.7955) knots 0 0 0 0 1 1 1 1
  spline S190 degree 3 poles (-18.3712, -32.7955) (-17.6268, -32.7955) (-16.9858, -32.8022) (-16.9476, -32.809) knots 0 0 0 0 1 1 1 1
  spline S191 degree 3 poles (-16.9476, -32.809) (-16.8509, -32.8292) (-16.6979, -32.9641) (-16.6485, -33.0743) knots 0 0 0 0 1 1 1 1
  spline S192 degree 3 poles (-16.6485, -33.0743) (-16.608, -33.162) (-16.6057, -33.2677) (-16.6057, -35.0467) knots 0 0 0 0 1 1 1 1
  spline S193 degree 3 poles (-16.6057, -35.0467) (-16.6057, -36.8391) (-16.608, -36.9291) (-16.6462, -36.9628) knots 0 0 0 0 1 1 1 1
  spline S194 degree 3 poles (-16.6462, -36.9628) (-16.6844, -36.9965) (-16.8171, -37.001) (-18.0968, -37.001) knots 0 0 0 0 1 1 1 1
  spline S195 degree 3 poles (-18.0968, -37.001) (-19.4664, -37.001) (-19.5069, -37.0033) (-19.5294, -37.0438) knots 0 0 0 0 1 1 1 1
  spline S196 degree 3 poles (-19.5294, -37.0438) (-19.5406, -37.0685) (-19.5519, -37.2192) (-19.5519, -37.3811) knots 0 0 0 0 1 1 1 1
  spline S197 degree 3 poles (-19.5519, -37.3811) (-19.5519, -37.6577) (-19.5496, -37.6757) (-19.5024, -37.7072) knots 0 0 0 0 1 1 1 1
  spline S198 degree 3 poles (-19.5024, -37.7072) (-19.4574, -37.7387) (-19.282, -37.7432) (-18.0563, -37.7432) knots 0 0 0 0 1 1 1 1
  spline S199 degree 3 poles (-18.0563, -37.7432) (-16.9993, -37.7432) (-16.653, -37.7499) (-16.6327, -37.7702) knots 0 0 0 0 1 1 1 1
  spline S200 degree 3 poles (-16.6327, -37.7702) (-16.6125, -37.7904) (-16.6057, -38.2694) (-16.6057, -39.7852) knots 0 0 0 0 1 1 1 1
  spline S201 degree 3 poles (-16.6057, -39.7852) (-16.6057, -41.9982) (-16.5967, -41.8655) (-16.7587, -41.9892) knots 0 0 0 0 1 1 1 1
  line L44 (-16.7587, -41.9892) -> (-16.8374, -42.0499)
  line L45 (-16.8374, -42.0499) -> (-18.4589, -42.0567)
  spline S202 degree 3 poles (-18.4589, -42.0567) (-19.9139, -42.0634) (-20.0939, -42.0589) (-20.2221, -42.0252) knots 0 0 0 0 1 1 1 1
  spline S203 degree 3 poles (-20.2221, -42.0252) (-20.4807, -41.9577) (-20.7438, -41.7418) (-20.8675, -41.5012) knots 0 0 0 0 1 1 1 1
  spline S204 degree 3 poles (-20.8675, -41.5012) (-20.899, -41.4382) (-20.917, -41.3865) (-20.9102, -41.3865) knots 0 0 0 0 1 1 1 1
  spline S205 degree 3 poles (-20.9102, -41.3865) (-20.9012, -41.3865) (-20.908, -41.3707) (-20.9237, -41.3528) knots 0 0 0 0 1 1 1 1
  spline S206 degree 3 poles (-20.9237, -41.3528) (-20.9372, -41.3348) (-20.944, -41.31) (-20.9372, -41.2988) knots 0 0 0 0 1 1 1 1
  spline S207 degree 3 poles (-20.9372, -41.2988) (-20.9282, -41.2875) (-20.9305, -41.2718) (-20.9417, -41.265) knots 0 0 0 0 1 1 1 1
  spline S208 degree 3 poles (-20.9417, -41.265) (-20.9507, -41.2605) (-20.962, -41.2111) (-20.9642, -41.1571) knots 0 0 0 0 1 1 1 1
  spline S209 degree 3 poles (-20.9642, -41.1571) (-20.971, -41.0222) (-20.9934, -40.8377) (-21.0069, -40.8198) knots 0 0 0 0 1 1 1 1
  spline S210 degree 3 poles (-21.0069, -40.8198) (-21.0114, -40.8085) (-21.1216, -40.8018) (-21.2521, -40.8018) knots 0 0 0 0 1 1 1 1
  line L46 (-21.2521, -40.8018) -> (-21.4882, -40.8018)
  line L47 (-21.4882, -40.8018) -> (-21.4747, -40.9322)
  spline S211 degree 3 poles (-21.4747, -40.9322) (-21.468, -41.0019) (-21.4477, -41.328) (-21.4297, -41.6564) knots 0 0 0 0 1 1 1 1
  spline S212 degree 3 poles (-21.4297, -41.6564) (-21.4118, -41.9847) (-21.3893, -42.3311) (-21.3825, -42.4278) knots 0 0 0 0 1 1 1 1
  line L48 (-21.3825, -42.4278) -> (-21.369, -42.6009)
  line L49 (-21.369, -42.6009) -> (-16.9408, -42.6009)
  line L50 (-16.9408, -42.6009) -> (-12.5126, -42.6009)
  line L51 (-12.5126, -42.6009) -> (-12.5126, -42.511)
extrude "Extrude6" cut sketch "Sketch5" along normal blind 1 contours S0 S1 S2 S3 S4 S5 S6 S7 S8 S9 S10 L0 L1 S11 S12 S13 S14 S15 S16 S17 S18 S19 L2 L3 L4 L5 S20 S21 | L6 L7 S22 S23 S24 S25 S26 S27 S28 S29 S30 S31 S32 S33 S34 S35 S36 S37 S38 S39 S40 S41 S42 L8 L9 L10 L11 S43 S44 S45 S46 S47 S48 S49 S50 S51 S52 S53 S54 S55 S56 S57 L12 L13 S58 S59 S60 S61 S62 S63 S64 S65 S66 S67 S68 S69 S70 S71 S72 S73 S74 S75 S76 S77 S78 S79 S80 S81 S82 S83 S84 S85 S86 S87 S88 S89 S90 S91 S92 S93 S94 S95 S96 S97 S98 S99 S100 S101 S102 S103 L14 L15 S104 S105 S106 S107 S108 S109 S110 S111 L16 L17 L18 L19 | S130 S131 S132 S133 L20 L21 L22 L23 S134 S135 S136 S137 S138 S139 S140 S141 S142 S143 S144 S145 S146 S147 S148 L24 L25 S149 S150 S151 S152 S153 S154 S155 L26 L27 L28 L29 L30 L31 L32 L33 S156 S157 S158 S159 S160 S161 S162 S163 S164 S165 S166 S167 S168 S169 S170 S171 S172 S173 S174 S175 S176 S177 S178 S179 S180 S181 S182 L34 L35 S183 | L36 L37 S184 S185 L38 L39 L40 L41 L42 L43 S186 S187 S188 S189 S190 S191 S192 S193 S194 S195 S196 S197 S198 S199 S200 S201 L44 L45 S202 S203 S204 S205 S206 S207 S208 S209 S210 L46 L47 S211 S212 L48 L49 L50 L51
equation "d4 = 8 mm - 0.125 mm"
